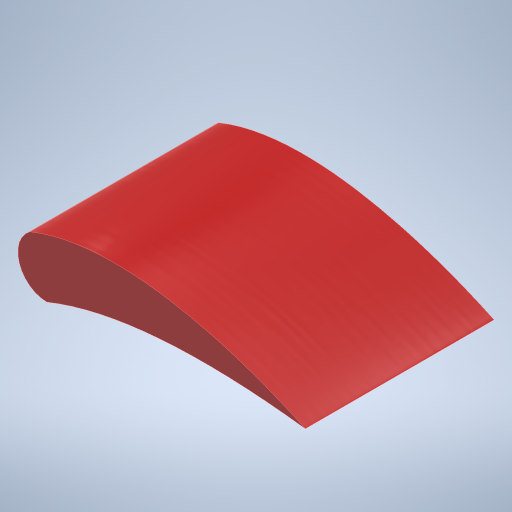
# Autodesk Inventor part: PALE
Saved by Autodesk Inventor 2024.2 (Build 282272000, 272)
## iProperties
Created: 2025-07-15
Part Number: PALE
Material: Generic
Document SubType Name: Modeling
Designer: KABONGO
Density: 1 g/cm^3
Appearance: Red
Author: KABONGO
Autodesk Inventor part; units mm, degrees
ref_plane "YZ Plane" through (0, 0, 0) normal (1, 0, 0) x (0, 1, 0)
ref_plane "XZ Plane" through (0, 0, 0) normal (0, 1, 0) x (-1, 0, 0)
ref_plane "XY Plane" through (0, 0, 0) normal (0, 0, 1) x (1, 0, 0)
sketch "Sketch1" plane through (0, 0, 0) normal (0, 0, 1) x (1, 0, 0)
  arc A0 (-17.8812, 52.2471) -> (4.7414, -18.3459) centre (4.7414, 20.5755) ccw
  line L0 (-17.8812, 52.2471) -> (141.2167, 116.6849) construction
  line L1 (141.2167, 116.6849) -> (349.4431, 7.9295) construction
  line L2 (349.4431, 7.9295) -> (352.6574, 7.9295) construction
  spline S0 degree 3 poles (-17.8812, 52.2471) (141.2167, 116.6849) (349.4431, 7.9295) (352.6574, 7.9295) knots 1 1 1 1 2 2 2 2
  line L3 (4.7414, -18.3459) -> (135.9231, 34.7853) construction
  line L4 (135.9231, 34.7853) -> (352.6574, 7.9295) construction
  spline S1 degree 2 poles (4.7414, -18.3459) (135.9231, 34.7853) (352.6574, 7.9295) knots 1 1 1 2 2 2
  point P0 (0, 0)
  constraints: 2 point on circle, 1 centre point, 1 horizontal, 6 other
extrude "Extrusion1" add sketch "Sketch1" along normal blind 254
body "Solid1"
